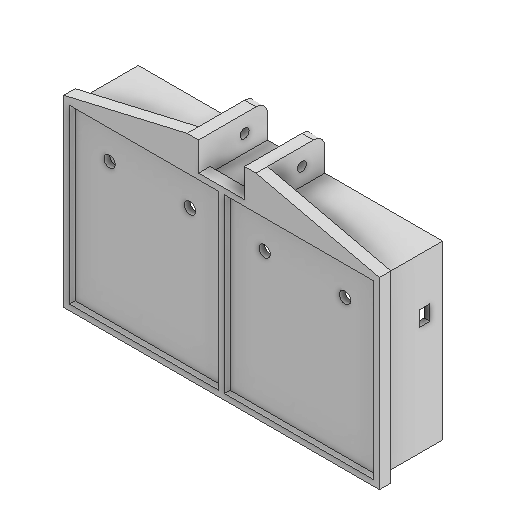
# Autodesk Inventor part: PlacaExcavacion
Saved by Autodesk Inventor 2025.2 (Build 292293000, 293)
## iProperties
Created: 2025-07-31
Part Number: PlacaExcavacion
Material: Genérico
Document SubType Name: Modeling
Designer: Triax_Tray
Density: 1 g/cm^3
Appearance: Valor por defecto
Author: Triax_Tray
Autodesk Inventor part; units mm, degrees
ref_plane "YZ Plane" through (0, 0, 0) normal (1, 0, 0) x (0, 1, 0)
ref_plane "XZ Plane" through (0, 0, 0) normal (0, 1, 0) x (-1, 0, 0)
ref_plane "XY Plane" through (0, 0, 0) normal (0, 0, 1) x (1, 0, 0)
sketch "Boceto1" plane through (0, 0, 0) normal (0, 0, 1) x (1, 0, 0)
  line L0 (0, 0) -> (130, 0)
  line L1 (130, 0) -> (130, 150)
  line L2 (130, 150) -> (0, 150)
  line L3 (0, 150) -> (0, 0)
  line L4 (135, 150) -> (135, 0)
  line L5 (135, 150) -> (265, 150)
  line L6 (265, 150) -> (265, 0)
  line L7 (265, 0) -> (135, 0)
  line L8 (270, 150) -> (270, 0)
  line L9 (270, 150) -> (270, 155)
  line L10 (270, 155) -> (0, 155)
  line L11 (0, 155) -> (-5, 155)
  line L12 (-5, 155) -> (-5, 0)
  line L13 (-5, 0) -> (-5, -5)
  line L14 (-5, -5) -> (270, -5)
  line L15 (270, 0) -> (270, -5)
  constraints: 32 end point, 6 perpendicular, 4 horizontal, 2 vertical, 1 point on line
extrude "Extrusión1" add sketch "Boceto1" along normal blind 5
sketch "Boceto2" plane through (0, 0, 0) normal (0, 0, -1) x (-1, 0, 0)
  line L0 (-270, 155) -> (5, 155) projected
  line L1 (-135, 150) -> (-265, 150) projected
  line L2 (-265, 150) -> (-265, 0) projected
  line L3 (-270, -5) -> (-270, 155) projected
  line L4 (5, -5) -> (-270, -5) projected
  line L5 (5, 155) -> (5, -5) projected
  line L6 (-270, 155) -> (5, 155)
  line L7 (5, 155) -> (5, -5)
  line L8 (0, 0) -> (0, 150) projected
  line L9 (-270, 155) -> (-270, -5)
  line L10 (-270, -5) -> (5, -5)
  constraints: 8 end point, 2 parallel, 1 collinear, 1 horizontal
extrude "Extrusión2" add sketch "Boceto2" along normal blind 5
sketch "Boceto3" plane through (0, 0, 0) normal (0, 0, 1) x (1, 0, 0)
  line L0 (0, 0) -> (0, 150) projected
  circle A0 centre (30, 120) radius 5
  circle A1 centre (100, 120) radius 5
  line L1 (130, 150) -> (132.5, 150)
  circle A2 centre (235, 120) radius 5
  circle A3 centre (165, 120) radius 5
  dimension "d17" = 10
  constraints: 4 centre point, 2 end point
  measures "d17" diameter of A0
extrude "Extrusión3" cut sketch "Boceto3" against normal blind 20
sketch "Boceto5" plane through (0, 0, -5) normal (0, 0, -1) x (-1, 0, 0)
  line L0 (5, 155) -> (-270, 155) projected
  circle A0 centre (-165, 120) radius 5 projected
  circle A1 centre (-100, 120) radius 5 projected
  circle A2 centre (-235, 120) radius 5 projected
  circle A3 centre (-30, 120) radius 5 projected
  line L1 (5, 155) -> (-270, 155) projected
  line L2 (-270, 155) -> (-270, -5) projected
  line L3 (-270, -5) -> (5, -5) projected
  line L4 (5, -5) -> (5, 155) projected
  line L5 (0, 0) -> (0, 150) projected
  line L6 (-270, 155) -> (5, 155) projected
  line L7 (-270, 155) -> (-270, -5) projected
  line L8 (-132.5, -5) -> (-122.5, -5) construction
  line L9 (-132.5, 5) -> (-5, 5)
  line L10 (0, 150) -> (-130, 150) projected
  line L11 (-260, 5) -> (-260, 140)
  line L12 (-5, 145) -> (-5, 5)
  line L13 (-5, 5) -> (-260, 5)
  line L14 (-260, 5) -> (-260, 140.9585)
  line L15 (-256.5, 145) -> (-5, 145)
  line L16 (-5, 145) -> (-5, 5)
  line L17 (-5, 5) -> (-260, 5)
  line L18 (-260, 5) -> (-260, 140.9585)
  line L19 (-265, 145) -> (-265, 5)
  line L20 (-130, 0) -> (0, 0) projected
  line L21 (-265, 150) -> (-265, 0) projected
  line L22 (-265, 145) -> (-265, 150)
  line L23 (-265, 150) -> (0, 150)
  line L24 (0, 0) -> (0, 150)
  line L25 (0, 0) -> (-265, 0)
  line L26 (-265, 0) -> (-265, 150)
  line L27 (-256.5, 145) -> (-132.5, 145)
  line L28 (-260, 5) -> (-132.5, 5)
  line L29 (-5, 145) -> (-5, 75)
  line L30 (-5, 145) -> (65, 145) construction
  line L31 (-260, 145) -> (-260, 75)
  line L32 (-1.5, 142.9793) -> (-5, 140.9585)
  line L33 (-5, 140.9585) -> (-8.5, 142.9793)
  line L34 (-8.5, 142.9793) -> (-8.5, 147.0207)
  line L35 (-8.5, 147.0207) -> (-5, 149.0415)
  line L36 (-5, 149.0415) -> (-1.5, 147.0207)
  line L37 (-1.5, 147.0207) -> (-1.5, 142.9793)
  line L38 (-1.5, 72.9793) -> (-5, 70.9585)
  line L39 (-5, 70.9585) -> (-8.5, 72.9793)
  line L40 (-8.5, 72.9793) -> (-8.5, 77.0207)
  line L41 (-8.5, 77.0207) -> (-5, 79.0415)
  line L42 (-5, 79.0415) -> (-1.5, 77.0207)
  line L43 (-1.5, 77.0207) -> (-1.5, 72.9793)
  line L44 (-1.5, 2.9793) -> (-5, 0.9585)
  line L45 (-5, 0.9585) -> (-8.5, 2.9793)
  line L46 (-8.5, 2.9793) -> (-8.5, 7.0207)
  line L47 (-8.5, 7.0207) -> (-5, 9.0415)
  line L48 (-5, 9.0415) -> (-1.5, 7.0207)
  line L49 (-1.5, 7.0207) -> (-1.5, 2.9793)
  line L50 (-129, 2.9793) -> (-132.5, 0.9585)
  line L51 (-132.5, 0.9585) -> (-136, 2.9793)
  line L52 (-136, 2.9793) -> (-136, 7.0207)
  line L53 (-136, 7.0207) -> (-132.5, 9.0415)
  line L54 (-132.5, 9.0415) -> (-129, 7.0207)
  line L55 (-129, 7.0207) -> (-129, 2.9793)
  line L56 (-256.5, 2.9793) -> (-260, 0.9585)
  line L57 (-260, 0.9585) -> (-263.5, 2.9793)
  line L58 (-263.5, 2.9793) -> (-263.5, 7.0207)
  line L59 (-263.5, 7.0207) -> (-260, 9.0415)
  line L60 (-260, 9.0415) -> (-256.5, 7.0207)
  line L61 (-256.5, 7.0207) -> (-256.5, 2.9793)
  line L62 (-256.5, 72.9793) -> (-260, 70.9585)
  line L63 (-260, 70.9585) -> (-263.5, 72.9793)
  line L64 (-263.5, 72.9793) -> (-263.5, 77.0207)
  line L65 (-263.5, 77.0207) -> (-260, 79.0415)
  line L66 (-260, 79.0415) -> (-256.5, 77.0207)
  line L67 (-256.5, 77.0207) -> (-256.5, 72.9793)
  line L68 (-256.5, 142.9793) -> (-260, 140.9585)
  line L69 (-260, 140.9585) -> (-263.5, 142.9793)
  line L70 (-263.5, 142.9793) -> (-263.5, 147.0207)
  line L71 (-263.5, 147.0207) -> (-260, 149.0415)
  line L72 (-260, 149.0415) -> (-256.5, 147.0207)
  line L73 (-256.5, 147.0207) -> (-256.5, 142.9793)
  line L74 (-129, 142.9793) -> (-132.5, 140.9585)
  line L75 (-132.5, 140.9585) -> (-136, 142.9793)
  line L76 (-136, 142.9793) -> (-136, 147.0207)
  line L77 (-136, 147.0207) -> (-132.5, 149.0415)
  line L78 (-132.5, 149.0415) -> (-129, 147.0207)
  line L79 (-129, 147.0207) -> (-129, 142.9793)
  circle A4 centre (-260, 145) radius 5
  circle A5 centre (-132.5, 145) radius 5
  circle A6 centre (-5, 145) radius 5
  circle A7 centre (-5, 75) radius 5
  circle A8 centre (-5, 5) radius 5
  circle A9 centre (-132.5, 5) radius 5
  circle A10 centre (-260, 5) radius 5
  circle A11 centre (-260, 75) radius 5
  line L80 (-260, 145) -> (-256.5, 145) construction
  line L81 (-255, 145) -> (-189.5, 145) construction
  point P0 (-1.5, 145)
  point P1 (-1.5, 75)
  point P2 (-1.5, 5)
  point P3 (-129, 5)
  point P4 (-256.5, 5)
  point P5 (-256.5, 75)
  point P6 (-129, 145)
  point P7 (-10, 145)
  point P8 (-5, 140)
  point P9 (-5, 80)
  point P10 (-5, 70)
  point P11 (-5, 10)
  point P12 (-10, 5)
  point P13 (-127.5, 5)
  point P14 (-137.5, 5)
  point P15 (-255, 5)
  point P16 (-260, 10)
  point P17 (-260, 70)
  point P18 (-260, 80)
  point P19 (-255, 145)
  point P20 (-137.5, 145)
  point P21 (-127.5, 145)
  dimension "d79" = 127.5
  dimension "d80" = 127.5
  dimension "d83" = 70
  dimension "d84" = 90
  dimension "d86" = 70
  dimension "d89" = 10
  dimension "d90" = 10
  dimension "d91" = 10
  dimension "d92" = 10
  dimension "d93" = 10
  dimension "d94" = 10
  dimension "d95" = 10
  dimension "d96" = 10
  constraints: 142 end point, 13 coincident, 10 midpoint, 8 centre point, 8 point on line, 6 horizontal, 5 collinear, 5 parallel, 3 perpendicular, 2 point on circle, 1 vertical, 104 other
  measures "d79" distance of L31.start L27.end
  measures "d80" distance of L28.start L9.start
  measures "d83" distance of L29.start L29.end
  measures "d84" angle of L29 L30
  measures "d86" distance of L31.start L31.end
  measures "d89" diameter of A4
  measures "d90" diameter of A5
  measures "d91" diameter of A6
  measures "d92" diameter of A7
  measures "d93" diameter of A8
  measures "d94" diameter of A9
  measures "d95" diameter of A10
  measures "d96" diameter of A11
extrude "Extrusion5" add sketch "Boceto5" along normal blind 10 contours L20 A8 L5 | A8 L12 A7 L5 | A8 L9 L46 L45 L44 L49 L48 L12 | L20 L25 A9 L9 A8 | A7 L12 A6 L5 | A7 L12 L38 L43 L42 | L12 L47 L46 L9 A8 | A6 L10 L5 | A6 L12 L32 L37 L36 L35 L34 L15 | L12 L41 L40 L39 A7 | L48 L49 L44 L45 L46 L9 L12 | L12 L9 L46 L47 | L25 A10 L13 A9 | A9 L13 L52 L51 L50 L55 L9 | L9 L55 L54 L53 L52 L13 A9 | A6 L15 A5 L23 L10 | A6 L15 L34 L33 L12 | L42 L43 L38 L12 | L12 L39 L40 L41 | L25 L21 A10 | A10 L11 L59 L58 L57 L56 L61 L13 | L55 L50 L51 L52 L13 L9 | L9 L13 L52 L53 L54 L55 | L33 L34 L15 L12 | L12 L15 L34 L35 L36 L37 L32 | L19 A11 L11 A10 | L13 L61 L60 L11 A10 | A5 L15 A4 L23 | A5 L15 L79 L78 L77 L76 | A5 L15 L76 L75 L74 L79 | L19 A4 L11 A11 | A11 L11 L65 L64 L63 | L61 L56 L57 L58 L59 L11 L13 | L13 L11 L60 L61 | A4 L21 L23 | A4 L15 L73 L72 L71 L70 L69 L14 | L79 L74 L75 L76 L15 | L15 L76 L77 L78 L79 | A11 L11 L62 L67 L66 | A4 L14 L68 L73 L15 | L66 L67 L62 L11 | L11 L63 L64 L65 | L73 L68 L69 L70 L71 L72
sketch "Sketch16" plane through (0, 0, -15) normal (0, 0, -1) x (-1, 0, 0)
  line L0 (-265, 0) -> (0, 0) projected
  line L1 (0, 0) -> (0, 150) projected
  line L2 (0, 150) -> (-265, 150) projected
  line L3 (-265, 150) -> (-265, 0) projected
  arc A0 (-10, 145) -> (-5, 140) centre (-5, 145) ccw projected
  line L4 (-5, 140) -> (-5, 80) projected
  arc A1 (-5, 80) -> (-5, 70) centre (-5, 75) ccw projected
  line L5 (-5, 70) -> (-5, 10) projected
  arc A2 (-5, 10) -> (-10, 5) centre (-5, 5) ccw projected
  line L6 (-10, 5) -> (-127.5, 5) projected
  arc A3 (-127.5, 5) -> (-137.5, 5) centre (-132.5, 5) ccw projected
  line L7 (-137.5, 5) -> (-255, 5) projected
  arc A4 (-255, 5) -> (-260, 10) centre (-260, 5) ccw projected
  line L8 (-260, 10) -> (-260, 70) projected
  arc A5 (-260, 70) -> (-260, 80) centre (-260, 75) ccw projected
  line L9 (-260, 80) -> (-260, 140) projected
  arc A6 (-260, 140) -> (-255, 145) centre (-260, 145) ccw projected
  line L10 (-255, 145) -> (-137.5, 145) projected
  arc A7 (-137.5, 145) -> (-127.5, 145) centre (-132.5, 145) ccw projected
  line L11 (-127.5, 145) -> (-10, 145) projected
  circle A8 centre (-132.5, 5) radius 2.5
  circle A9 centre (-5, 5) radius 2.5
  circle A10 centre (-5, 75) radius 2.5
  circle A11 centre (-5, 145) radius 2.5
  circle A12 centre (-132.5, 145) radius 2.5
  circle A13 centre (-260, 145) radius 2.5
  circle A14 centre (-260, 75) radius 2.5
  circle A15 centre (-260, 5) radius 2.5
  dimension "d190" = 5
  dimension "d191" = 5
  dimension "d192" = 5
  dimension "d193" = 5
  dimension "d194" = 5
  dimension "d195" = 5
  dimension "d196" = 5
  dimension "d197" = 5
  constraints: 8 centre point, 8 coincident
  measures "d190" diameter of A8
  measures "d191" diameter of A9
  measures "d192" diameter of A10
  measures "d193" diameter of A11
  measures "d194" diameter of A12
  measures "d195" diameter of A13
  measures "d196" diameter of A14
  measures "d197" diameter of A15
extrude "Extrusion13" add sketch "Sketch16" along normal blind 15
sketch "Sketch17" plane through (0, 0, -30) normal (0, 0, -1) x (-1, 0, 0)
  line L0 (0, 0) -> (0, 150) projected
  line L1 (0, 150) -> (-265, 150) projected
  line L2 (-265, 150) -> (-265, 0) projected
  line L3 (-265, 0) -> (0, 0) projected
  circle A0 centre (-260, 5) radius 2.5 projected
  circle A1 centre (-260, 75) radius 2.5 projected
  circle A2 centre (-260, 145) radius 2.5 projected
  circle A3 centre (-132.5, 145) radius 2.5 projected
  circle A4 centre (-5, 145) radius 2.5 projected
  circle A5 centre (-5, 75) radius 2.5 projected
  circle A6 centre (-5, 5) radius 2.5 projected
  circle A7 centre (-132.5, 5) radius 2.5 projected
  arc A8 (-10, 145) -> (-5, 140) centre (-5, 145) ccw projected
  line L4 (-5, 140) -> (-5, 80) projected
  arc A9 (-5, 80) -> (-5, 70) centre (-5, 75) ccw projected
  line L5 (-5, 70) -> (-5, 10) projected
  arc A10 (-5, 10) -> (-10, 5) centre (-5, 5) ccw projected
  line L6 (-10, 5) -> (-127.5, 5) projected
  arc A11 (-127.5, 5) -> (-137.5, 5) centre (-132.5, 5) ccw projected
  line L7 (-137.5, 5) -> (-255, 5) projected
  arc A12 (-255, 5) -> (-260, 10) centre (-260, 5) ccw projected
  line L8 (-260, 10) -> (-260, 70) projected
  arc A13 (-260, 70) -> (-260, 80) centre (-260, 75) ccw projected
  line L9 (-260, 80) -> (-260, 140) projected
  arc A14 (-260, 140) -> (-255, 145) centre (-260, 145) ccw projected
  line L10 (-255, 145) -> (-137.5, 145) projected
  arc A15 (-137.5, 145) -> (-127.5, 145) centre (-132.5, 145) ccw projected
  line L11 (-127.5, 145) -> (-10, 145) projected
  circle A16 centre (-132.5, 5) radius 3.875
  line L12 (-132.5, 1.125) -> (-135.8558, 3.0625)
  line L13 (-135.8558, 3.0625) -> (-135.8558, 6.9375)
  line L14 (-135.8558, 6.9375) -> (-132.5, 8.875)
  line L15 (-132.5, 8.875) -> (-129.1442, 6.9375)
  line L16 (-129.1442, 6.9375) -> (-129.1442, 3.0625)
  line L17 (-129.1442, 3.0625) -> (-132.5, 1.125)
  circle A17 centre (-260, 5) radius 3.875
  line L18 (-260, 1.125) -> (-263.3558, 3.0625)
  line L19 (-263.3558, 3.0625) -> (-263.3558, 6.9375)
  line L20 (-263.3558, 6.9375) -> (-260, 8.875)
  line L21 (-260, 8.875) -> (-256.6442, 6.9375)
  line L22 (-256.6442, 6.9375) -> (-256.6442, 3.0625)
  line L23 (-256.6442, 3.0625) -> (-260, 1.125)
  circle A18 centre (-260, 75) radius 3.875
  line L24 (-260, 71.125) -> (-263.3558, 73.0625)
  line L25 (-263.3558, 73.0625) -> (-263.3558, 76.9375)
  line L26 (-263.3558, 76.9375) -> (-260, 78.875)
  line L27 (-260, 78.875) -> (-256.6442, 76.9375)
  line L28 (-256.6442, 76.9375) -> (-256.6442, 73.0625)
  line L29 (-256.6442, 73.0625) -> (-260, 71.125)
  circle A19 centre (-260, 145) radius 3.875
  line L30 (-260, 141.125) -> (-263.3558, 143.0625)
  line L31 (-263.3558, 143.0625) -> (-263.3558, 146.9375)
  line L32 (-263.3558, 146.9375) -> (-260, 148.875)
  line L33 (-260, 148.875) -> (-256.6442, 146.9375)
  line L34 (-256.6442, 146.9375) -> (-256.6442, 143.0625)
  line L35 (-256.6442, 143.0625) -> (-260, 141.125)
  circle A20 centre (-132.5, 145) radius 3.875
  line L36 (-132.5, 141.125) -> (-135.8558, 143.0625)
  line L37 (-135.8558, 143.0625) -> (-135.8558, 146.9375)
  line L38 (-135.8558, 146.9375) -> (-132.5, 148.875)
  line L39 (-132.5, 148.875) -> (-129.1442, 146.9375)
  line L40 (-129.1442, 146.9375) -> (-129.1442, 143.0625)
  line L41 (-129.1442, 143.0625) -> (-132.5, 141.125)
  circle A21 centre (-5, 145) radius 3.875
  line L42 (-5, 141.125) -> (-8.3558, 143.0625)
  line L43 (-8.3558, 143.0625) -> (-8.3558, 146.9375)
  line L44 (-8.3558, 146.9375) -> (-5, 148.875)
  line L45 (-5, 148.875) -> (-1.6442, 146.9375)
  line L46 (-1.6442, 146.9375) -> (-1.6442, 143.0625)
  line L47 (-1.6442, 143.0625) -> (-5, 141.125)
  circle A22 centre (-5, 75) radius 3.875
  line L48 (-5, 71.125) -> (-8.3558, 73.0625)
  line L49 (-8.3558, 73.0625) -> (-8.3558, 76.9375)
  line L50 (-8.3558, 76.9375) -> (-5, 78.875)
  line L51 (-5, 78.875) -> (-1.6442, 76.9375)
  line L52 (-1.6442, 76.9375) -> (-1.6442, 73.0625)
  line L53 (-1.6442, 73.0625) -> (-5, 71.125)
  circle A23 centre (-5, 5) radius 3.875
  line L54 (-5, 1.125) -> (-8.3558, 3.0625)
  line L55 (-8.3558, 3.0625) -> (-8.3558, 6.9375)
  line L56 (-8.3558, 6.9375) -> (-5, 8.875)
  line L57 (-5, 8.875) -> (-1.6442, 6.9375)
  line L58 (-1.6442, 6.9375) -> (-1.6442, 3.0625)
  line L59 (-1.6442, 3.0625) -> (-5, 1.125)
  dimension "d200" = 7.75
  dimension "d201" = 7.75
  dimension "d202" = 7.75
  dimension "d203" = 7.75
  dimension "d204" = 7.75
  dimension "d205" = 7.75
  dimension "d206" = 7.75
  dimension "d207" = 7.75
  constraints: 96 end point, 16 coincident, 8 vertical alignment, 120 other
extrude "Extrusion14" add sketch "Sketch17" along normal blind 3.25 contours L3 L2 L1 L0 | A16 L16 | L15 A16 | A16 L17 | L14 A16 | A16 L12 | L13 A16 | A17 L22 | L21 A17 | A17 L23 | L20 A17 | A17 L18 | L19 A17 | A18 L28 | L27 A18 | A18 L29 | L26 A18 | A18 L24 | L25 A18 | A19 L34 | L33 A19 | A19 L35 | L32 A19 | A19 L30 | L31 A19 | A20 L40 | L39 A20 | A20 L41 | L38 A20 | A20 L36 | L37 A20 | A21 L46 | L45 A21 | A21 L47 | L44 A21 | A21 L42 | L43 A21 | A22 L52 | L51 A22 | A22 L53 | L50 A22 | A22 L48 | L49 A22 | A23 L58 | L57 A23 | A23 L59 | L56 A23 | A23 L54 | L55 A23
sketch "Sketch18" plane through (0, 0, -33.25) normal (0, 0, -1) x (-1, 0, 0)
  line L0 (0, 150) -> (-265, 150) projected
  line L1 (-265, 150) -> (-265, 0) projected
  line L2 (-265, 0) -> (0, 0) projected
  line L3 (0, 0) -> (0, 150) projected
  line L4 (-1.6442, 6.9375) -> (-1.6442, 3.0625) projected
  line L5 (-1.6442, 3.0625) -> (-5, 1.125) projected
  line L6 (-5, 1.125) -> (-8.3558, 3.0625) projected
  line L7 (-8.3558, 3.0625) -> (-8.3558, 6.9375) projected
  line L8 (-8.3558, 6.9375) -> (-5, 8.875) projected
  line L9 (-5, 8.875) -> (-1.6442, 6.9375) projected
  line L10 (-1.6442, 76.9375) -> (-1.6442, 73.0625) projected
  line L11 (-1.6442, 73.0625) -> (-5, 71.125) projected
  line L12 (-5, 71.125) -> (-8.3558, 73.0625) projected
  line L13 (-8.3558, 73.0625) -> (-8.3558, 76.9375) projected
  line L14 (-8.3558, 76.9375) -> (-5, 78.875) projected
  line L15 (-5, 78.875) -> (-1.6442, 76.9375) projected
  line L16 (-1.6442, 146.9375) -> (-1.6442, 143.0625) projected
  line L17 (-1.6442, 143.0625) -> (-5, 141.125) projected
  line L18 (-5, 141.125) -> (-8.3558, 143.0625) projected
  line L19 (-8.3558, 143.0625) -> (-8.3558, 146.9375) projected
  line L20 (-8.3558, 146.9375) -> (-5, 148.875) projected
  line L21 (-5, 148.875) -> (-1.6442, 146.9375) projected
  line L22 (-129.1442, 146.9375) -> (-129.1442, 143.0625) projected
  line L23 (-129.1442, 143.0625) -> (-132.5, 141.125) projected
  line L24 (-132.5, 141.125) -> (-135.8558, 143.0625) projected
  line L25 (-135.8558, 143.0625) -> (-135.8558, 146.9375) projected
  line L26 (-135.8558, 146.9375) -> (-132.5, 148.875) projected
  line L27 (-132.5, 148.875) -> (-129.1442, 146.9375) projected
  line L28 (-256.6442, 146.9375) -> (-256.6442, 143.0625) projected
  line L29 (-256.6442, 143.0625) -> (-260, 141.125) projected
  line L30 (-260, 141.125) -> (-263.3558, 143.0625) projected
  line L31 (-263.3558, 143.0625) -> (-263.3558, 146.9375) projected
  line L32 (-263.3558, 146.9375) -> (-260, 148.875) projected
  line L33 (-260, 148.875) -> (-256.6442, 146.9375) projected
  line L34 (-256.6442, 76.9375) -> (-256.6442, 73.0625) projected
  line L35 (-256.6442, 73.0625) -> (-260, 71.125) projected
  line L36 (-260, 71.125) -> (-263.3558, 73.0625) projected
  line L37 (-263.3558, 73.0625) -> (-263.3558, 76.9375) projected
  line L38 (-263.3558, 76.9375) -> (-260, 78.875) projected
  line L39 (-260, 78.875) -> (-256.6442, 76.9375) projected
  line L40 (-256.6442, 6.9375) -> (-256.6442, 3.0625) projected
  line L41 (-256.6442, 3.0625) -> (-260, 1.125) projected
  line L42 (-260, 1.125) -> (-263.3558, 3.0625) projected
  line L43 (-263.3558, 3.0625) -> (-263.3558, 6.9375) projected
  line L44 (-263.3558, 6.9375) -> (-260, 8.875) projected
  line L45 (-260, 8.875) -> (-256.6442, 6.9375) projected
  line L46 (-129.1442, 6.9375) -> (-129.1442, 3.0625) projected
  line L47 (-129.1442, 3.0625) -> (-132.5, 1.125) projected
  line L48 (-132.5, 1.125) -> (-135.8558, 3.0625) projected
  line L49 (-135.8558, 3.0625) -> (-135.8558, 6.9375) projected
  line L50 (-135.8558, 6.9375) -> (-132.5, 8.875) projected
  line L51 (-132.5, 8.875) -> (-129.1442, 6.9375) projected
  arc A0 (-10, 145) -> (-5, 140) centre (-5, 145) ccw projected
  line L52 (-5, 140) -> (-5, 80) projected
  arc A1 (-5, 80) -> (-5, 70) centre (-5, 75) ccw projected
  line L53 (-5, 70) -> (-5, 10) projected
  arc A2 (-5, 10) -> (-10, 5) centre (-5, 5) ccw projected
  line L54 (-10, 5) -> (-127.5, 5) projected
  arc A3 (-127.5, 5) -> (-137.5, 5) centre (-132.5, 5) ccw projected
  line L55 (-137.5, 5) -> (-255, 5) projected
  arc A4 (-255, 5) -> (-260, 10) centre (-260, 5) ccw projected
  line L56 (-260, 10) -> (-260, 70) projected
  arc A5 (-260, 70) -> (-260, 80) centre (-260, 75) ccw projected
  line L57 (-260, 80) -> (-260, 140) projected
  arc A6 (-260, 140) -> (-255, 145) centre (-260, 145) ccw projected
  line L58 (-255, 145) -> (-137.5, 145) projected
  arc A7 (-137.5, 145) -> (-127.5, 145) centre (-132.5, 145) ccw projected
  line L59 (-127.5, 145) -> (-10, 145) projected
  circle A8 centre (-5, 145) radius 2.05
  circle A9 centre (-5, 75) radius 2.05
  circle A10 centre (-5, 5) radius 2.05
  circle A11 centre (-132.5, 5) radius 2.5 projected
  circle A12 centre (-132.5, 5) radius 2.05
  circle A13 centre (-260, 5) radius 2.05
  circle A14 centre (-260, 75) radius 2.05
  circle A15 centre (-260, 145) radius 2.05
  circle A16 centre (-132.5, 145) radius 2.05
  dimension "d210" = 4.1
  dimension "d211" = 4.1
  dimension "d212" = 4.1
  dimension "d213" = 4.1
  dimension "d214" = 4.1
  dimension "d215" = 4.1
  dimension "d216" = 4.1
  dimension "d217" = 4.1
  constraints: 8 centre point, 8 coincident
  measures "d210" diameter of A8
  measures "d211" diameter of A9
  measures "d212" diameter of A10
  measures "d213" diameter of A12
  measures "d214" diameter of A13
  measures "d215" diameter of A14
  measures "d216" diameter of A15
  measures "d217" diameter of A16
extrude "Extrusion15" add sketch "Sketch18" along normal blind 21.75 contours L3 L2 L1 L0 | L4 L5 L6 L7 L8 L9 | L10 L11 L12 L13 L14 L15 | L16 L17 L18 L19 L20 L21 | L22 L23 L24 L25 L26 L27 | L28 L29 L30 L31 L32 L33 | L34 L35 L36 L37 L38 L39 | L40 L41 L42 L43 L44 L45 | L46 L47 L48 L49 L50 L51 | A11
sketch "Sketch19" plane through (0, 0, -5) normal (0, 0, -1) x (-1, 0, 0)
  line L0 (-265, 150) -> (-265, 0) projected
  line L1 (-265, 0) -> (0, 0) projected
  line L2 (0, 0) -> (0, 150) projected
  line L3 (0, 150) -> (-265, 150) projected
  circle A0 centre (-5, 5) radius 2.05 projected
  circle A1 centre (-5, 75) radius 2.05 projected
  circle A2 centre (-5, 145) radius 2.05 projected
  circle A3 centre (-132.5, 145) radius 2.05 projected
  arc A4 (-10, 145) -> (-5, 140) centre (-5, 145) ccw projected
  line L4 (-5, 140) -> (-5, 80) projected
  arc A5 (-5, 80) -> (-5, 70) centre (-5, 75) ccw projected
  line L5 (-5, 70) -> (-5, 10) projected
  arc A6 (-5, 10) -> (-10, 5) centre (-5, 5) ccw projected
  line L6 (-10, 5) -> (-127.5, 5) projected
  arc A7 (-127.5, 5) -> (-137.5, 5) centre (-132.5, 5) ccw projected
  line L7 (-137.5, 5) -> (-255, 5) projected
  arc A8 (-255, 5) -> (-260, 10) centre (-260, 5) ccw projected
  line L8 (-260, 10) -> (-260, 70) projected
  arc A9 (-260, 70) -> (-260, 80) centre (-260, 75) ccw projected
  line L9 (-260, 80) -> (-260, 140) projected
  arc A10 (-260, 140) -> (-255, 145) centre (-260, 145) ccw projected
  line L10 (-255, 145) -> (-137.5, 145) projected
  arc A11 (-137.5, 145) -> (-127.5, 145) centre (-132.5, 145) ccw projected
  line L11 (-127.5, 145) -> (-10, 145) projected
  circle A12 centre (-132.5, 5) radius 2.05 projected
  circle A13 centre (-260, 5) radius 2.05 projected
  circle A14 centre (-260, 75) radius 2.05 projected
  circle A15 centre (-260, 145) radius 2.05 projected
  circle A16 centre (-240, 95) radius 2
  circle A17 centre (-135, 95) radius 2
  circle A18 centre (-135, 45) radius 2
  circle A19 centre (-240, 45) radius 2
  circle A20 centre (-240, 95) radius 4
  circle A21 centre (-135, 95) radius 4
  circle A22 centre (-135, 45) radius 4
  circle A23 centre (-240, 45) radius 4
  dimension "d227" = 4
  dimension "d229" = 4
  dimension "d231" = 4
  dimension "d233" = 4
  dimension "d234" = 8
  dimension "d235" = 8
  dimension "d236" = 8
  dimension "d237" = 8
  constraints: 8 centre point, 4 coincident
  measures "d227" diameter of A16
  measures "d229" diameter of A17
  measures "d231" diameter of A18
  measures "d233" diameter of A19
  measures "d234" diameter of A20
  measures "d235" diameter of A21
  measures "d236" diameter of A22
  measures "d237" diameter of A23
extrude "Extrusion16" add sketch "Sketch19" along normal blind 10 contours A20 | A21 | A22 | A23
thread "Thread5" size "M4x0.7" class "6H" standard "ANSI Metric M Profile" full length
thread "Thread6" size "M4x0.7" class "6H" standard "ANSI Metric M Profile" full length
thread "Thread7" size "M4x0.7" class "6H" standard "ANSI Metric M Profile" full length
thread "Thread8" size "M4x0.7" class "6H" standard "ANSI Metric M Profile" full length
fillet "Fillet1" radius 2 1 edges at (244, 95, -5)
fillet "Fillet2" radius 2 16 edges at (260, 110, -5) (255, 75, -5) (260, 40, -5) (196.25, 145, -5) (256.4645, 141.4645, -5) (132.5, 140, -5) (68.75, 145, -5) (8.5355, 141.4645, -5) (5, 110, -5) (68.75, 5, -5) (132.5, 10, -5) (196.25, 5, -5) (256.4645, 8.5355, -5) (5, 40, -5) (8.5355, 8.5355, -5) (10, 75, -5)
fillet "Fillet3" radius 2 3 edges at (244, 45, -5) (139, 45, -5) (139, 95, -5)
sketch "Sketch20" plane through (265, 0, -5) normal (1, 0, 0) x (0, 0, -1)
  line L0 (0, 0) -> (0, 150) projected
  line L1 (0, 0) -> (50, 0) projected
  line L2 (50, 150) -> (50, 0) projected
  line L3 (0, 150) -> (50, 150) projected
  line L4 (30, 95) -> (30, 108.2)
  line L5 (-5, 150) -> (-5, 0) projected
  line L6 (30, 108.2) -> (39, 108.2)
  line L7 (39, 108.2) -> (39, 95)
  line L8 (39, 95) -> (30, 95)
  dimension "d253" = 13.2
  dimension "d254" = 9
  dimension "d255" = 13.2
  constraints: 8 end point, 1 horizontal, 1 parallel, 1 perpendicular
  measures "d253" distance of L4.start L4.end
  measures "d254" distance of L4.end L6.end
  measures "d255" distance of L6.end L7.end
extrude "Extrusion17" cut sketch "Sketch20" against normal blind 10 contours L4 L6 L7 L8
sketch "Sketch21" plane through (0, 0, -5) normal (0, -1, 0) x (1, 0, 0)
  line L0 (134.55, -50) -> (130.45, -50) projected
  circle A0 centre (112.5, -30) radius 7.6
  point P0 (0, 5)
  dimension "d262" = 15.2
  constraints: 1 centre point
  measures "d262" diameter of A0
extrude "Extrusion18" cut sketch "Sketch21" against normal blind 20
sketch "Sketch22" plane through (0, 150, -5) normal (0, 1, 0) x (1, 0, 0)
  line L0 (265, 0) -> (0, 0) projected
  line L1 (265, 0) -> (265, 50) projected
  line L2 (0, 50) -> (265, 50) projected
  line L3 (0, 0) -> (0, 50) projected
  line L4 (-5, 0) -> (-5, -10) projected
  line L5 (270, -10) -> (-5, -10) projected
  line L6 (270, -10) -> (270, 0) projected
  line L7 (-5, 0) -> (270, 0) projected
  line L8 (0, 50) -> (132.5, 50)
  line L9 (132.5, 50) -> (162.5, 50)
  line L10 (162.5, 50) -> (162.5, -10)
  line L11 (162.5, 50) -> (152.5, 50)
  line L12 (152.5, 50) -> (152.5, -10)
  line L13 (152.5, -10) -> (162.5, -10)
  line L14 (132.5, 50) -> (102.5, 50)
  line L15 (102.5, 50) -> (102.5, -10)
  line L16 (102.5, -10) -> (112.5, -10)
  line L17 (270, -10) -> (-5, -10) projected
  line L18 (112.5, -10) -> (112.5, 50)
  line L19 (112.5, 50) -> (102.5, 50)
  line L20 (152.5, 50) -> (162.5, 50)
  point P0 (0, -5)
  point P1 (152.5, 0)
  point P2 (162.5, 0)
  point P3 (112.5, 0)
  point P4 (102.5, 0)
  dimension "d265" = 132.5
  dimension "d266" = 30
  dimension "d267" = 10
  dimension "d268" = 30
  dimension "d269" = 10
  constraints: 24 end point, 8 point on line, 4 perpendicular, 3 collinear, 1 midpoint
  measures "d265" distance of L2.start L8.end
  measures "d266" distance of L8.end L9.end
  measures "d267" distance of L9.end L11.end
  measures "d268" distance of L8.end L14.end
  measures "d269" distance of L15.end L16.end
extrude "Extrusion19" add sketch "Sketch22" along normal blind 30 contours L0 L12 L2 L10 | L0 L15 L2 L18
sketch "Sketch23" plane through (-5, 155, 5) normal (0, 1, 0) x (1, 0, 0)
  line L0 (275, 0) -> (0, 0) projected
  line L1 (117.5, 10) -> (157.5, 10) projected
  line L2 (107.5, 10) -> (117.5, 10) projected
  line L3 (157.5, 10) -> (167.5, 10) projected
  line L4 (167.5, 10) -> (275, 10) projected
  line L5 (0, 10) -> (107.5, 10) projected
  line L6 (107.5, 10) -> (107.5, 0)
  line L7 (117.5, 10) -> (117.5, 0)
  line L8 (107.5, 0) -> (117.5, 0)
  line L9 (157.5, 10) -> (167.5, 10)
  line L10 (260, 12) -> (142.5, 12) projected
  line L11 (167.5, 10) -> (167.5, 0)
  line L12 (157.5, 10) -> (157.5, 0)
  line L13 (157.5, 0) -> (167.5, 0)
  point P0 (5, 5)
  constraints: 14 end point, 4 perpendicular, 4 point on line, 2 collinear, 1 parallel
extrude "Extrusion20" add sketch "Sketch23" along normal blind 25 contours L0 L12 L3 L11 | L0 L6 L2 L7
sketch "Sketch24" plane through (0, 0, -5) normal (0, 0, -1) x (-1, 0, 0)
  line L0 (5, 155) -> (-102.5, 155) projected
  line L1 (-102.5, 150) -> (-102.5, 180) projected
  line L2 (-112.5, 180) -> (-102.5, 180) projected
  line L3 (-162.5, 155) -> (-270, 155) projected
  line L4 (-162.5, 180) -> (-152.5, 180) projected
  line L5 (-162.5, 150) -> (-162.5, 180) projected
  line L6 (5, 155) -> (-102.5, 180)
  line L7 (-270, 155) -> (-162.5, 180)
  point P0 (0, 0)
  constraints: 4 end point
extrude "Extrusion21" add sketch "Sketch24" against normal blind 10
sketch "Sketch25" plane through (102.5, 150, -55) normal (-1, 0, 0) x (0, 0, 1)
  line L0 (50, 0) -> (50, 30) projected
  line L1 (0, 30) -> (50, 30) projected
  line L2 (0, 0) -> (0, 30) projected
  line L3 (50, 0) -> (0, 0) projected
  line L4 (0, 0) -> (20, 0)
  circle A0 centre (20, 15) radius 4
  point P0 (55, -150)
  dimension "d278" = 8
  constraints: 2 end point, 1 centre point, 1 point on line
  measures "d278" diameter of A0
extrude "Extrusion22" cut sketch "Sketch25" against normal blind 80 contours A0
fillet "Fillet4" radius 10 2 edges at (107.5, 180, -55) (157.5, 180, -55)
sketch "Sketch27" plane through (0, 0, -5) normal (0, 0, -1) x (-1, 0, 0)
  circle A0 centre (-135, 95) radius 2 projected
  line L0 (-11.7082, 7) -> (-125.7918, 7) projected
  line L1 (-20.1726, 95) -> (-20.1726, 85)
  line L2 (-20.1726, 95) -> (-30.1726, 95)
  line L3 (-20.1726, 95) -> (-10.1726, 95) construction
  line L4 (-13.1015, 102.0711) -> (-30.1726, 95)
  line L5 (-13.1015, 102.0711) -> (-20.1726, 85)
  line L6 (-20.1726, 35) -> (-30.1726, 35)
  line L7 (-20.1726, 35) -> (-20.1726, 45)
  line L8 (-20.1726, 35) -> (-10.1726, 35) construction
  line L9 (-20.1726, 45) -> (-13.1015, 27.9289)
  line L10 (-30.1726, 35) -> (-13.1015, 27.9289)
  line L11 (-112.1726, 95) -> (-102.1726, 95)
  line L12 (-112.1726, 95) -> (-112.1726, 85)
  line L13 (-112.1726, 95) -> (-102.1726, 95) construction
  line L14 (-119.2436, 102.0711) -> (-112.1726, 85)
  line L15 (-102.1726, 95) -> (-119.2436, 102.0711)
  point P0 (0, 0)
  dimension "d285" = 92
  constraints: 30 end point, 3 horizontal
  measures "d285" distance of L1.start L11.start
extrude "Extrusion23" add sketch "Sketch27" along normal blind 13 contours L2 L4 L5 L1 | L7 L9 L10 L6 | L12 L14 L15 L11
draft "FaceDraft1" angle 20 pull direction (0, 0, -1) faces at (18.7918, 99.714, -13.6667) fixed edges at (21.637, 98.5355, -5)
draft "FaceDraft2" angle 21 pull direction (0, 0, -1) faces at (17.2884, 91.963, -13.6667) fixed edges at (14.5659, 98.5355, -5) (18.1015, 90, -5)
draft "FaceDraft3" angle 21 pull direction (0, 0, -1) faces at (24.4822, 32.643, -9.3333) fixed edges at (21.637, 31.4645, -5)
draft "FaceDraft4" angle 21 pull direction (0, 0, -1) faces at (17.335, 38.1497, -13.6667) fixed edges at (14.5659, 31.4645, -5) (18.1015, 40, -5)
draft "FaceDraft5" angle 21 pull direction (0, 0, -1) faces at (23.5584, 96.3807, -8.4495) fixed edges at (25.1726, 97.0711, -5) (16.637, 100.6066, -5)
draft "FaceDraft6" angle 21 pull direction (0, 0, -1) faces at (116.8866, 96.3807, -13.6667) fixed edges at (115.7081, 93.5355, -5)
draft "FaceDraft7" angle 21 pull direction (0, 0, -1) faces at (109.0229, 97.8375, -13.6667) fixed edges at (115.7081, 100.6066, -5) (107.1726, 97.0711, -5)
sketch "Sketch28" plane through (0, 0, -5) normal (0, 0, -1) x (-1, 0, 0)
  line L0 (-20.1726, 45) -> (-20.1726, 35) projected
  line L1 (-30.1726, 35) -> (-20.1726, 35) projected
  line L2 (-20.1726, 85) -> (-20.1726, 95) projected
  line L3 (-30.1726, 95) -> (-20.1726, 95) projected
  line L4 (-102.1726, 95) -> (-112.1726, 95) projected
  line L5 (-112.1726, 85) -> (-112.1726, 95) projected
  line L6 (-112.1726, 95) -> (-112.1726, 35)
  line L7 (-112.1726, 35) -> (-120.1726, 35)
  circle A0 centre (-116.1726, 35) radius 4
  circle A1 centre (-116.1726, 35) radius 2
  line L8 (-116.1726, 31) -> (-120.1726, 31)
  point P0 (0, 0)
  dimension "d314" = 8
  dimension "d315" = 4
  constraints: 6 end point, 2 centre point, 2 point on circle, 1 coincident, 1 horizontal, 1 midpoint, 1 parallel, 1 tangent, 1 vertical
  measures "d314" distance of L6.end L7.end
  measures "d315" diameter of A1
extrude "Extrusion24" add sketch "Sketch28" along normal blind 5 contours A0 L7 A1 | L7 A1 A0
thread "Thread9" size "M4x0.7" class "6H" standard "ANSI Metric M Profile" full length
fillet "Fillet5" radius 2 1 edges at (120.1726, 35, -5)
